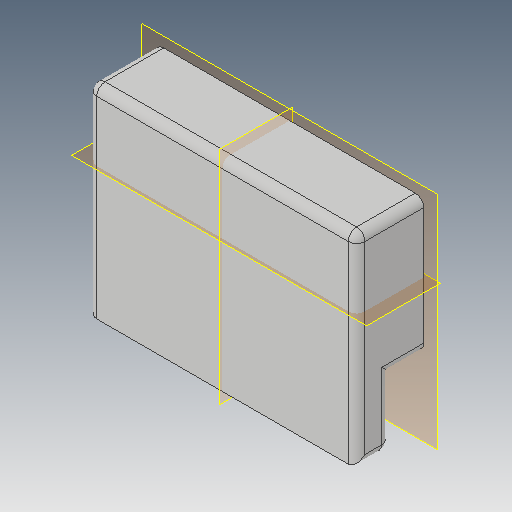
# Autodesk Inventor part: handle
Saved by Autodesk Inventor 2017 (Build 210142000, 142)
## iProperties
Created: 2018-11-28
Part Number: handle
Material: Generic
Document SubType Name: Modeling
Designer: jpb34
Density: 1 g/cm^3
Appearance: Default
Author: jpb34
Autodesk Inventor part; units mm, degrees
sketch "Sketch1" plane through (0, 0, 0) normal (0, 0, 1) x (1, 0, 0)
  line L0 (-47.625, 26.0649) -> (47.625, 26.0649)
  line L1 (50.8, 22.8899) -> (50.8, -21.5601)
  line L2 (47.625, -24.7351) -> (-47.625, -24.7351)
  line L3 (-50.8, -21.5601) -> (-50.8, 22.8899)
  arc A0 (-47.625, 26.0649) -> (-50.8, 22.8899) centre (-47.625, 22.8899) ccw
  arc A1 (-50.8, -21.5601) -> (-47.625, -24.7351) centre (-47.625, -21.5601) ccw
  arc A2 (47.625, -24.7351) -> (50.8, -21.5601) centre (47.625, -21.5601) ccw
  arc A3 (50.8, 22.8899) -> (47.625, 26.0649) centre (47.625, 22.8899) ccw
  point P0 (0, 0)
  point P1 (-50.8, 26.0649)
  point P2 (50.8, -24.7351)
  point P3 (50.8, 26.0649)
  dimension "d0" = 101.6
  dimension "d1" = 50.8
  dimension "d2" = 3.175
  dimension "d10" = 50.8
  constraints: 8 end point, 8 point on circle, 8 tangent, 6 point on line, 4 centre point, 3 equal radius, 2 parallel, 1 horizontal, 1 perpendicular
  measures "d0" distance of point (-50.8, 26.065) point (50.8, 26.065)
  measures "d1" distance of point (50.8, 26.065) point (50.8, -24.735)
  measures "d2" radius of A0
  measures "d10" distance from line of point (0, 0) L3
extrude "Extrusion1" add sketch "Sketch1" along normal blind 12.7
sketch "Sketch2" plane through (0, 0, 12.7) normal (0, 0, 1) x (1, 0, 0)
  line L0 (-47.625, 26.0649) -> (47.625, 26.0649)
  line L1 (50.8, 22.8899) -> (50.8, -50.1351)
  line L2 (50.8, -50.1351) -> (-50.8, -50.1351)
  line L3 (-50.8, -50.1351) -> (-50.8, 22.8899)
  line L4 (47.625, 26.0649) -> (-47.625, 26.0649) projected
  arc A0 (-47.625, 26.0649) -> (-50.8, 22.8899) centre (-47.625, 22.8899) ccw
  arc A1 (50.8, 22.8899) -> (47.625, 26.0649) centre (47.625, 22.8899) ccw
  point P0 (0, 0)
  point P1 (50.8, 26.0649)
  dimension "d5" = 76.2
  dimension "d6" = 0
  dimension "d7" = 101.6
  dimension "d8" = 50.8
  dimension "d9" = 3.175
  dimension "d11" = 3.175
  constraints: 8 end point, 4 point on circle, 4 tangent, 2 centre point, 2 parallel, 2 point on line, 1 horizontal, 1 perpendicular
  measures "d5" distance of point (50.8, 26.065) L1.end
  measures "d6" distance between parallel lines of L4 L0
  measures "d7" distance of L1.end L2.end
  measures "d8" distance from line of point (0, 0) L1
  measures "d9" radius of A0
  measures "d11" radius of A1
extrude "Extrusion2" add sketch "Sketch2" along normal blind 12.7
fillet "Fillet1" radius 3.175 1 edges at (0, -50.1351, 12.7)
fillet "Fillet2" radius 3.175 8 edges at (50.8, -50.1351, 20.6375) (50.8, -49.2051, 13.6299) (50.8, -34.2601, 12.7) (-49.8701, 25.135, 25.4) (-50.8, -13.6226, 25.4) (49.8701, 25.135, 25.4) (50.8, -13.6226, 25.4) (0, 26.0649, 25.4)
body "Solid1"
